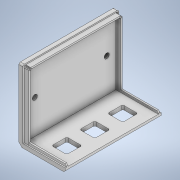
# Autodesk Inventor part: sUPORTE
Saved by Autodesk Inventor 2022 (Build 260153000, 153)
## iProperties
Created: 2022-12-13
Part Number: sUPORTE
Material: Genérico
Document SubType Name: Modeling
Designer: gugarauj07
Density: 1 g/cm^3
Appearance: Padrão
Author: gugarauj07
Autodesk Inventor part; units mm, degrees
ref_plane "YZ Plane" through (0, 0, 0) normal (1, 0, 0) x (0, 1, 0)
ref_plane "XZ Plane" through (0, 0, 0) normal (0, 1, 0) x (-1, 0, 0)
ref_plane "XY Plane" through (0, 0, 0) normal (0, 0, 1) x (1, 0, 0)
sketch "Esboço1" plane through (0, 0, 0) normal (1, 0, 0) x (0, 1, 0)
  line L0 (40.5, 60) -> (-42.5, 60)
  line L1 (-42.5, 60) -> (-42.5, -60)
  line L2 (-42.5, -60) -> (40.5, -60)
  line L3 (42.5, -58) -> (42.5, 58)
  line L4 (-42.5, 60) -> (42.5, -60) construction
  arc A0 (42.5, 58) -> (40.5, 60) centre (40.5, 58) ccw
  arc A1 (40.5, -60) -> (42.5, -58) centre (40.5, -58) ccw
  point P0 (0, 0)
  dimension "d0" = 85
  dimension "d1" = 120
  dimension "d4" = 2
  constraints: 10 end point, 4 point on circle, 4 tangent, 2 centre point, 2 parallel, 2 point on line, 1 equal radius, 1 horizontal, 1 midpoint, 1 perpendicular
  measures "d0" distance of L4.end L1.end
  measures "d1" distance of L0.end L1.end
  measures "d4" radius of A0
extrude "Extrusão1" add sketch "Esboço1" along normal blind 5
sketch "Esboço2" plane through (5, 0, 0) normal (1, 0, 0) x (0, 0, -1)
  line L0 (-60, 40.5) -> (-60, -42.5) projected
  line L1 (-60, -42.5) -> (-58.5, -42.5)
  line L2 (-60, -42.5) -> (60, -42.5) projected
  line L3 (60, -42.5) -> (58.5, -42.5)
  arc A0 (-58, 42.5) -> (-60, 40.5) centre (-58, 40.5) ccw projected
  line L4 (-58, 42.5) -> (-58, 41)
  line L5 (-58.5, -42.5) -> (-56.5, -42.5)
  line L6 (-56.5, -42.5) -> (-56.5, 37)
  line L7 (-56.5, 41) -> (-56.5, 41)
  line L8 (-58.5, 39) -> (-58.5, -42.5)
  line L9 (58.5, -42.5) -> (56.5, -42.5)
  line L10 (56.5, -42.5) -> (56.5, 37)
  line L11 (56.5, 41) -> (56.5, 41)
  line L12 (58.5, 39) -> (58.5, -42.5)
  line L13 (-56.5, 41) -> (56.5, 41)
  line L14 (54.5, 39) -> (-54.5, 39)
  arc A1 (-56.5, 41) -> (-58.5, 39) centre (-56.5, 39) ccw
  arc A2 (-54.5, 39) -> (-56.5, 37) centre (-54.5, 37) ccw
  arc A3 (58.5, 39) -> (56.5, 41) centre (56.5, 39) ccw
  arc A4 (56.5, 37) -> (54.5, 39) centre (54.5, 37) ccw
  point P0 (0, 0)
  point P1 (-58.5, 41)
  point P2 (58.5, 41)
  dimension "d7" = 1.5
  dimension "d8" = 1.5
  dimension "d9" = 1.5
  dimension "d10" = 2
  dimension "d11" = 2
  dimension "d13" = 2
  constraints: 26 end point, 9 point on line, 8 point on circle, 8 tangent, 5 parallel, 4 centre point, 3 equal radius, 3 horizontal, 2 perpendicular, 1 vertical
  measures "d7" distance of L0.end L1.end
  measures "d8" distance of L2.end L3.end
  measures "d9" distance of L4.start L4.end
  measures "d10" distance of point (-58.5, 41) L7.start
  measures "d11" distance of L11.start point (58.5, 41)
  measures "d13" radius of A1
extrude "Extrusão2" add sketch "Esboço2" along normal blind 6 contours L8 A1 L13 A3 L12 L2 L10 A4 L14 A2 L6
sketch "Esboço3" plane through (11, 0, 0) normal (1, 0, 0) x (0, 0, -1)
  circle A0 centre (-57, 39.5) radius 1.6
  circle A1 centre (57, 39.5) radius 1.6
  point P0 (0, 0)
  dimension "d18" = 3.2
  constraints: 2 centre point
  measures "d18" diameter of A0
hole "Furo1" at (11, 39.5, 57) direction (-1, 0, 0) diameter 3.302 depth 40 tip angle 118 thread size "8-32 UNC" class "2B" standard "ANSI Unified Screw Threads"
hole "Furo2" at (11, 39.5, -57) direction (-1, 0, 0) diameter 3.302 depth 40 tip angle 118 thread size "8-32 UNC" class "2B" standard "ANSI Unified Screw Threads"
sketch "Esboço4" plane through (5, 0, 0) normal (1, 0, 0) x (0, 0, -1)
  line L0 (-60, -42.5) -> (60, -42.5) projected
  line L1 (-60, -42.5) -> (60, -42.5)
  line L2 (60, -42.5) -> (60, -47.5)
  line L3 (60, -47.5) -> (-60, -47.5)
  line L4 (-60, -47.5) -> (-60, -42.5)
  point P0 (0, 0)
  point P1 (60, -42.5)
  dimension "d33" = 5
  constraints: 8 end point, 2 parallel, 1 horizontal, 1 perpendicular
  measures "d33" distance of L1.end L2.end
extrude "Extrusão3" add sketch "Esboço4" against normal blind 5
sketch "Esboço5" plane through (5, 0, 0) normal (1, 0, 0) x (0, 0, -1)
  line L0 (-60, 40.5) -> (-60, -47.5) projected
  line L1 (60, 40.5) -> (60, -47.5) projected
  line L2 (-60, -47.5) -> (60, -47.5)
  line L3 (60, -47.5) -> (60, -42.5)
  line L4 (60, -42.5) -> (-60, -42.5)
  line L5 (-60, -42.5) -> (-60, -47.5)
  point P0 (0, 0)
  point P1 (60, -47.5)
  dimension "d36" = 5
  constraints: 8 end point, 2 parallel, 1 horizontal, 1 perpendicular, 1 point on line
  measures "d36" distance of L3.end L2.end
extrude "Extrusão4" add sketch "Esboço5" along normal blind 53.158
sketch "Esboço6" plane through (11, 0, 0) normal (1, 0, 0) x (0, 0, -1)
  line L0 (60, -42.5) -> (-60, -42.5) projected
  line L1 (-58.4844, -42.5) -> (-56.4844, -42.5)
  line L2 (-56.4844, -42.5) -> (-56.4844, -39.5)
  line L3 (-56.4844, -39.5) -> (-58.4844, -39.5)
  line L4 (-58.4844, -39.5) -> (-58.4844, -42.5)
  line L5 (56.5, 37) -> (56.5, -42.5) projected
  line L6 (58.5, 38.8102) -> (58.5, -42.5) projected
  line L7 (56.5, -42.5) -> (58.5, -42.5)
  line L8 (58.5, -42.5) -> (58.5, -39.5)
  line L9 (58.5, -39.5) -> (56.5, -39.5)
  line L10 (56.5, -39.5) -> (56.5, -42.5)
  point P0 (0, 0)
  dimension "d39" = 2
  dimension "d40" = 3
  dimension "d41" = 3
  constraints: 16 end point, 4 parallel, 2 horizontal, 2 perpendicular, 2 point on line
  measures "d39" distance of L3.end L2.end
  measures "d40" distance of L2.end L1.end
  measures "d41" distance of L8.end L7.end
extrude "Extrusão5" add sketch "Esboço6" along normal blind 47.158
chamfer "Chanfro1" distance 2 angle 45 2 edges at (58.158, -39.5, 57.4844) (58.158, -39.5, -57.5)
chamfer "Chanfro2" distance 4 angle 45 1 edges at (0, -47.5, 0)
chamfer "Chanfro3" distance 2 angle 45 1 edges at (58.158, -47.5, 0)
sketch "Esboço7" plane through (5, 0, 0) normal (1, 0, 0) x (0, 0, -1)
  circle A0 centre (-45, 0) radius 3
  circle A1 centre (45, 0) radius 3
  point P0 (0, 0)
  dimension "d61" = 6
  dimension "d62" = 6
  constraints: 2 centre point
  measures "d61" diameter of A0
  measures "d62" diameter of A1
hole "Furo3" at (5, 0, 45) direction (-1, 0, 0) diameter 6.4008 depth 22.931 tip angle 118 thread size "5/16-18 UNC" class "2B" standard "ANSI Unified Screw Threads"
hole "Furo4" at (5, 0, -45) direction (-1, 0, 0) diameter 6.4008 depth 22.931 tip angle 118 thread size "5/16-18 UNC" class "2B" standard "ANSI Unified Screw Threads"
sketch "Esboço8" plane through (5, -42.5, 56.5) normal (0, 1, 0) x (1, 0, 0)
  line L0 (0, 0) -> (0, 113) projected
  line L1 (0, 0) -> (30, 0)
  line L2 (0, 56.5) -> (0, 0)
  line L3 (22.5, 47) -> (37.5, 47)
  line L4 (39.5, 49) -> (39.5, 64)
  line L5 (37.5, 66) -> (22.5, 66)
  line L6 (20.5, 64) -> (20.5, 49)
  line L7 (20.5, 47) -> (39.5, 66) construction
  line L8 (39.5, 47) -> (20.5, 66) construction
  line L9 (22.5, 12) -> (37.5, 12)
  line L10 (39.5, 14) -> (39.5, 29)
  line L11 (37.5, 31) -> (22.5, 31)
  line L12 (20.5, 29) -> (20.5, 14)
  line L13 (20.5, 12) -> (39.5, 31) construction
  line L14 (39.5, 12) -> (20.5, 31) construction
  line L15 (22.5, 82) -> (37.5, 82)
  line L16 (39.5, 84) -> (39.5, 99)
  line L17 (37.5, 101) -> (22.5, 101)
  line L18 (20.5, 99) -> (20.5, 84)
  line L19 (20.5, 82) -> (39.5, 101) construction
  line L20 (39.5, 82) -> (20.5, 101) construction
  arc A0 (20.5, 14) -> (22.5, 12) centre (22.5, 14) ccw
  arc A1 (22.5, 31) -> (20.5, 29) centre (22.5, 29) ccw
  arc A2 (39.5, 29) -> (37.5, 31) centre (37.5, 29) ccw
  arc A3 (37.5, 12) -> (39.5, 14) centre (37.5, 14) ccw
  arc A4 (37.5, 47) -> (39.5, 49) centre (37.5, 49) ccw
  arc A5 (39.5, 64) -> (37.5, 66) centre (37.5, 64) ccw
  arc A6 (22.5, 66) -> (20.5, 64) centre (22.5, 64) ccw
  arc A7 (20.5, 49) -> (22.5, 47) centre (22.5, 49) ccw
  arc A8 (22.5, 101) -> (20.5, 99) centre (22.5, 99) ccw
  arc A9 (39.5, 99) -> (37.5, 101) centre (37.5, 99) ccw
  arc A10 (20.5, 84) -> (22.5, 82) centre (22.5, 84) ccw
  arc A11 (37.5, 82) -> (39.5, 84) centre (37.5, 84) ccw
  point P0 (-5, 56.5)
  dimension "d82" = 19
  dimension "d83" = 19
  dimension "d88" = 19
  dimension "d89" = 19
  dimension "d91" = 19
  dimension "d92" = 19
  dimension "d93" = 2
  dimension "d94" = 2
  constraints: 40 end point, 24 point on circle, 24 point on line, 24 tangent, 12 centre point, 10 equal radius, 6 parallel, 4 horizontal, 3 perpendicular
  measures "d82" distance of L8.end L7.end
  measures "d83" distance of L7.end L8.start
  measures "d88" distance of L14.end L13.end
  measures "d89" distance of L13.end L14.start
  measures "d91" distance of L20.end L19.end
  measures "d92" distance of L19.end L20.start
  measures "d93" radius of A0
  measures "d94" radius of A5
extrude "Extrusão6" cut sketch "Esboço8" against normal through all
